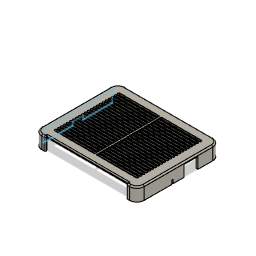
Grille (Autodesk Fusion 360 design; units mm, degrees)
Autodesk Fusion 360 part; units mm, degrees
sketch "Sketch1" plane through (0, 63.4, 0) normal (0, 1, 0) x (-1, 0, 0)
  line L0 (66.875, -54.475) -> (-66.875, -54.475)
  arc A0 (-68.875, -52.475) -> (-66.875, -54.475) centre (-66.875, -52.475) ccw
  line L1 (-68.875, -52.475) -> (-68.875, 52.475)
  arc A1 (-66.875, 54.475) -> (-68.875, 52.475) centre (-66.875, 52.475) ccw
  line L2 (-66.875, 54.475) -> (66.875, 54.475)
  arc A2 (68.875, 52.475) -> (66.875, 54.475) centre (66.875, 52.475) ccw
  line L3 (68.875, 52.475) -> (68.875, -52.475)
  arc A3 (66.875, -54.475) -> (68.875, -52.475) centre (66.875, -52.475) ccw
  line L4 (-66.4, -59.92) -> (66.4, -59.92)
  arc A4 (66.4, -59.92) -> (74.4, -51.92) centre (66.4, -51.92) ccw
  line L5 (74.4, -51.92) -> (74.4, 51.92)
  arc A5 (74.4, 51.92) -> (66.4, 59.92) centre (66.4, 51.92) ccw
  line L6 (66.4, 59.92) -> (-66.4, 59.92)
  arc A6 (-66.4, 59.92) -> (-74.4, 51.92) centre (-66.4, 51.92) ccw
  line L7 (-74.4, 51.92) -> (-74.4, -51.92)
  arc A7 (-74.4, -51.92) -> (-66.4, -59.92) centre (-66.4, -51.92) ccw
  line L8 (74.7, -51.92) -> (74.7, 51.92)
  arc A8 (74.7, 51.92) -> (66.4, 60.22) centre (66.4, 51.92) ccw
  line L9 (66.4, 60.22) -> (-66.4, 60.22)
  arc A9 (-66.4, 60.22) -> (-74.7, 51.92) centre (-66.4, 51.92) ccw
  line L10 (-74.7, 51.92) -> (-74.7, -51.92)
  arc A10 (-74.7, -51.92) -> (-66.4, -60.22) centre (-66.4, -51.92) ccw
  line L11 (-66.4, -60.22) -> (66.4, -60.22)
  arc A11 (66.4, -60.22) -> (74.7, -51.92) centre (66.4, -51.92) ccw
  line L12 (77.4, -51.92) -> (77.4, 51.92)
  arc A12 (77.4, 51.92) -> (66.4, 62.92) centre (66.4, 51.92) ccw
  line L13 (66.4, 62.92) -> (-66.4, 62.92)
  arc A13 (-66.4, 62.92) -> (-77.4, 51.92) centre (-66.4, 51.92) ccw
  line L14 (-77.4, 51.92) -> (-77.4, -51.92)
  arc A14 (-77.4, -51.92) -> (-66.4, -62.92) centre (-66.4, -51.92) ccw
  line L15 (-66.4, -62.92) -> (66.4, -62.92)
  arc A15 (66.4, -62.92) -> (77.4, -51.92) centre (66.4, -51.92) ccw
  dimension "d238" = 0.3
  dimension "d239" = 3
extrude "Extrude1" add sketch "Sketch1" against normal blind 17 contours L12 A12 L13 A13 L14 A14 L15 A15
extrude "Extrude2" add sketch "Sketch1" along normal blind 3 contours L0 A0 L1 A1 L2 A2 L3 A3 | L4 A4 L5 A5 L6 A6 L7 A7 | L8 A8 L9 A9 L10 A10 L11 A11 | L12 A12 L13 A13 L14 A14 L15 A15
sketch "Sketch2" plane through (0, 66.4, 0) normal (0, 1, 0) x (-1, 0, 0)
  line L0 (66.4, -59.92) -> (0, -59.92)
  line L1 (0, -59.92) -> (63, -59.92)
  line L2 (74.4, -51.92) -> (74.4, 0) construction
  line L3 (63, 0) -> (74.4, 0) construction
  line L4 (63, 0) -> (63, -48.5) construction
  line L5 (63, -48.5) -> (189, -48.5) construction
  line L6 (189, -48.5) -> (189, 48.5) construction
  line L7 (189, 48.5) -> (63, 48.5) construction
  line L8 (63, 48.5) -> (63, -48.5) construction
  line L9 (61.5, -47) -> (-61.5, -47)
  arc A0 (-61.5, -47) -> (-61.5, -50) centre (-61.5, -48.5) ccw
  line L10 (-61.5, -50) -> (61.5, -50)
  arc A1 (61.5, -50) -> (61.5, -47) centre (61.5, -48.5) ccw
  line L11 (63, -48.5) -> (-63, -48.5) construction
  line L12 (-61.5, -45.4762) -> (61.5, -45.4762)
  line L13 (61.5, -42.4762) -> (-61.5, -42.4762)
  arc A2 (61.5, -45.4762) -> (61.5, -42.4762) centre (61.5, -43.9762) ccw
  arc A3 (-61.5, -42.4762) -> (-61.5, -45.4762) centre (-61.5, -43.9762) ccw
  line L14 (-61.5, -40.9524) -> (61.5, -40.9524)
  line L15 (61.5, -37.9524) -> (-61.5, -37.9524)
  arc A4 (61.5, -40.9524) -> (61.5, -37.9524) centre (61.5, -39.4524) ccw
  arc A5 (-61.5, -37.9524) -> (-61.5, -40.9524) centre (-61.5, -39.4524) ccw
  line L16 (-61.5, -36.4286) -> (61.5, -36.4286)
  line L17 (61.5, -33.4286) -> (-61.5, -33.4286)
  arc A6 (61.5, -36.4286) -> (61.5, -33.4286) centre (61.5, -34.9286) ccw
  arc A7 (-61.5, -33.4286) -> (-61.5, -36.4286) centre (-61.5, -34.9286) ccw
  line L18 (-61.5, -31.9048) -> (61.5, -31.9048)
  line L19 (61.5, -28.9048) -> (-61.5, -28.9048)
  arc A8 (61.5, -31.9048) -> (61.5, -28.9048) centre (61.5, -30.4048) ccw
  arc A9 (-61.5, -28.9048) -> (-61.5, -31.9048) centre (-61.5, -30.4048) ccw
  line L20 (-61.5, -27.381) -> (61.5, -27.381)
  line L21 (61.5, -24.381) -> (-61.5, -24.381)
  arc A10 (61.5, -27.381) -> (61.5, -24.381) centre (61.5, -25.881) ccw
  arc A11 (-61.5, -24.381) -> (-61.5, -27.381) centre (-61.5, -25.881) ccw
  line L22 (-61.5, -22.8571) -> (61.5, -22.8571)
  line L23 (61.5, -19.8571) -> (-61.5, -19.8571)
  arc A12 (61.5, -22.8571) -> (61.5, -19.8571) centre (61.5, -21.3571) ccw
  arc A13 (-61.5, -19.8571) -> (-61.5, -22.8571) centre (-61.5, -21.3571) ccw
  line L24 (-61.5, -18.3333) -> (61.5, -18.3333)
  line L25 (61.5, -15.3333) -> (-61.5, -15.3333)
  arc A14 (61.5, -18.3333) -> (61.5, -15.3333) centre (61.5, -16.8333) ccw
  arc A15 (-61.5, -15.3333) -> (-61.5, -18.3333) centre (-61.5, -16.8333) ccw
  line L26 (-61.5, -13.8095) -> (61.5, -13.8095)
  line L27 (61.5, -10.8095) -> (-61.5, -10.8095)
  arc A16 (61.5, -13.8095) -> (61.5, -10.8095) centre (61.5, -12.3095) ccw
  arc A17 (-61.5, -10.8095) -> (-61.5, -13.8095) centre (-61.5, -12.3095) ccw
  line L28 (-61.5, -9.2857) -> (61.5, -9.2857)
  line L29 (61.5, -6.2857) -> (-61.5, -6.2857)
  arc A18 (61.5, -9.2857) -> (61.5, -6.2857) centre (61.5, -7.7857) ccw
  arc A19 (-61.5, -6.2857) -> (-61.5, -9.2857) centre (-61.5, -7.7857) ccw
  line L30 (-61.5, -4.7619) -> (61.5, -4.7619)
  line L31 (61.5, -1.7619) -> (-61.5, -1.7619)
  arc A20 (61.5, -4.7619) -> (61.5, -1.7619) centre (61.5, -3.2619) ccw
  arc A21 (-61.5, -1.7619) -> (-61.5, -4.7619) centre (-61.5, -3.2619) ccw
  line L32 (-61.5, -0.2381) -> (61.5, -0.2381)
  line L33 (61.5, 2.7619) -> (-61.5, 2.7619)
  arc A22 (61.5, -0.2381) -> (61.5, 2.7619) centre (61.5, 1.2619) ccw
  arc A23 (-61.5, 2.7619) -> (-61.5, -0.2381) centre (-61.5, 1.2619) ccw
  line L34 (-61.5, 4.2857) -> (61.5, 4.2857)
  line L35 (61.5, 7.2857) -> (-61.5, 7.2857)
  arc A24 (61.5, 4.2857) -> (61.5, 7.2857) centre (61.5, 5.7857) ccw
  arc A25 (-61.5, 7.2857) -> (-61.5, 4.2857) centre (-61.5, 5.7857) ccw
  line L36 (-61.5, 8.8095) -> (61.5, 8.8095)
  line L37 (61.5, 11.8095) -> (-61.5, 11.8095)
  arc A26 (61.5, 8.8095) -> (61.5, 11.8095) centre (61.5, 10.3095) ccw
  arc A27 (-61.5, 11.8095) -> (-61.5, 8.8095) centre (-61.5, 10.3095) ccw
  line L38 (-61.5, 13.3333) -> (61.5, 13.3333)
  line L39 (61.5, 16.3333) -> (-61.5, 16.3333)
  arc A28 (61.5, 13.3333) -> (61.5, 16.3333) centre (61.5, 14.8333) ccw
  arc A29 (-61.5, 16.3333) -> (-61.5, 13.3333) centre (-61.5, 14.8333) ccw
  line L40 (-61.5, 17.8571) -> (61.5, 17.8571)
  line L41 (61.5, 20.8571) -> (-61.5, 20.8571)
  arc A30 (61.5, 17.8571) -> (61.5, 20.8571) centre (61.5, 19.3571) ccw
  arc A31 (-61.5, 20.8571) -> (-61.5, 17.8571) centre (-61.5, 19.3571) ccw
  line L42 (-61.5, 22.381) -> (61.5, 22.381)
  line L43 (61.5, 25.381) -> (-61.5, 25.381)
  arc A32 (61.5, 22.381) -> (61.5, 25.381) centre (61.5, 23.881) ccw
  arc A33 (-61.5, 25.381) -> (-61.5, 22.381) centre (-61.5, 23.881) ccw
  line L44 (-61.5, 26.9048) -> (61.5, 26.9048)
  line L45 (61.5, 29.9048) -> (-61.5, 29.9048)
  arc A34 (61.5, 26.9048) -> (61.5, 29.9048) centre (61.5, 28.4048) ccw
  arc A35 (-61.5, 29.9048) -> (-61.5, 26.9048) centre (-61.5, 28.4048) ccw
  line L46 (-61.5, 31.4286) -> (61.5, 31.4286)
  line L47 (61.5, 34.4286) -> (-61.5, 34.4286)
  arc A36 (61.5, 31.4286) -> (61.5, 34.4286) centre (61.5, 32.9286) ccw
  arc A37 (-61.5, 34.4286) -> (-61.5, 31.4286) centre (-61.5, 32.9286) ccw
  line L48 (-61.5, 35.9524) -> (61.5, 35.9524)
  line L49 (61.5, 38.9524) -> (-61.5, 38.9524)
  arc A38 (61.5, 35.9524) -> (61.5, 38.9524) centre (61.5, 37.4524) ccw
  arc A39 (-61.5, 38.9524) -> (-61.5, 35.9524) centre (-61.5, 37.4524) ccw
  line L50 (-61.5, 40.4762) -> (61.5, 40.4762)
  line L51 (61.5, 43.4762) -> (-61.5, 43.4762)
  arc A40 (61.5, 40.4762) -> (61.5, 43.4762) centre (61.5, 41.9762) ccw
  arc A41 (-61.5, 43.4762) -> (-61.5, 40.4762) centre (-61.5, 41.9762) ccw
  line L52 (-61.5, 45) -> (61.5, 45)
  line L53 (61.5, 48) -> (-61.5, 48)
  arc A42 (61.5, 45) -> (61.5, 48) centre (61.5, 46.5) ccw
  arc A43 (-61.5, 48) -> (-61.5, 45) centre (-61.5, 46.5) ccw
  line L54 (0, -50) -> (1.5, -50)
  line L55 (1.5, -50) -> (-1.5, -50)
  line L56 (-1.5, -50) -> (-1.5, 48)
  line L57 (-1.5, 48) -> (1.5, 48)
  line L58 (1.5, 48) -> (1.5, -50)
  arc A44 (66.4, -62.92) -> (77.4, -51.92) centre (66.4, -51.92) ccw
  line L59 (77.4, -51.92) -> (77.4, 51.92)
  arc A45 (77.4, 51.92) -> (66.4, 62.92) centre (66.4, 51.92) ccw
  line L60 (66.4, 62.92) -> (-66.4, 62.92)
  arc A46 (-66.4, 62.92) -> (-77.4, 51.92) centre (-66.4, 51.92) ccw
  line L61 (-77.4, 51.92) -> (-77.4, -51.92)
  arc A47 (-77.4, -51.92) -> (-66.4, -62.92) centre (-66.4, -51.92) ccw
  line L62 (-66.4, -62.92) -> (66.4, -62.92)
  dimension "d244" = 63
  dimension "d246" = 48.5
  dimension "d247" = 126
  dimension "d248" = 97
  dimension "d249" = 126
  dimension "d250" = 3
  dimension "d253" = 0
  dimension "d254" = 95
  dimension "d257" = 1.5
  dimension "d258" = 3
  dimension "d259" = 98
  constraint coincident L0 L1.end
  constraint perpendicular L3 L4
  constraint horizontal L5
  constraint vertical L6
  constraint horizontal L7
  constraint vertical L8
  constraint tangent L9 A0
  constraint tangent A0 L10
  constraint parallel L9 L10
  constraint tangent L10 A1
  constraint tangent L9 A1
  constraint midpoint L4.end A1
  constraint midpoint A0 L11.end
  constraint perpendicular L4 L11
  constraint midpoint L10 L54.start
  constraint horizontal L54
  constraint horizontal L55
  constraint vertical L56
  constraint horizontal L57
  constraint vertical L58
  measures "d244" distance of L0.end L1.end
  measures "d246" distance of L3.start L4.end
  measures "d247" distance of L4.end L5.end
  measures "d248" distance of L4.end L7.end
  measures "d249" distance of L4.end L11.end
  measures "d250" diameter of A0
  measures "d257" distance of L54.start L54.end
  measures "d258" distance of L54.end L55.end
  measures "d259" distance of L54.end L57.end
extrude "Extrude3" cut sketch "Sketch2" against normal up to surface (3 mm away) contours L9 L10 A1 L58 | L9 A0 L10 L56 | L12 L13 A2 L58 | L12 L13 A3 L56 | L14 L15 A4 L58 | L14 L15 A5 L56 | L16 L17 A6 L58 | L16 L17 A7 L56 | L18 L19 A8 L58 | L18 L19 A9 L56 | L20 L21 A10 L58 | L20 L21 A11 L56 | L22 L23 A12 L58 | L22 L23 A13 L56 | L24 L25 A14 L58 | L24 L25 A15 L56 | L26 L27 A16 L58 | L26 L27 A17 L56 | L28 L29 A18 L58 | L28 L29 A19 L56 | L30 L31 A20 L58 | L30 L31 A21 L56 | L32 L33 A22 L58 | L32 L33 A23 L56 | L34 L35 A24 L58 | L34 L35 A25 L56 | L36 L37 A26 L58 | L36 L37 A27 L56 | L38 L39 A28 L58 | L38 L39 A29 L56 | L40 L41 A30 L58 | L40 L41 A31 L56 | L42 L43 A32 L58 | L42 L43 A33 L56 | L44 L45 A34 L58 | L44 L45 A35 L56 | L46 L47 A36 L58 | L46 L47 A37 L56 | L48 L49 A38 L58 | L48 L49 A39 L56 | L50 L51 A40 L58 | L50 L51 A41 L56 | L52 L53 A42 L58 | L52 L53 A43 L56
chamfer "Chamfer1" distance 0.7 angle 45 132 edges at (31.5, 63.4, 48) (63, 63.4, 46.5) (31.5, 63.4, 45) (31.5, 63.4, 43.4762) (63, 63.4, 41.9762) (31.5, 63.4, 40.4762) (31.5, 63.4, 38.9524) (63, 63.4, 37.4524) (31.5, 63.4, 35.9524) (31.5, 63.4, 34.4286) (63, 63.4, 32.9286) (31.5, 63.4, 31.4286) (31.5, 63.4, 29.9048) (63, 63.4, 28.4048) (31.5, 63.4, 26.9048) (31.5, 63.4, 25.381) (63, 63.4, 23.881) (31.5, 63.4, 22.381) (31.5, 63.4, 20.8571) (63, 63.4, 19.3571) (31.5, 63.4, 17.8571) (31.5, 63.4, 16.3333) (63, 63.4, 14.8333) (31.5, 63.4, 13.3333) (31.5, 63.4, 11.8095) (63, 63.4, 10.3095) (31.5, 63.4, 8.8095) (31.5, 63.4, 7.2857) (63, 63.4, 5.7857) (31.5, 63.4, 4.2857) (31.5, 63.4, 2.7619) (63, 63.4, 1.2619) (31.5, 63.4, -0.2381) (31.5, 63.4, -1.7619) (63, 63.4, -3.2619) (31.5, 63.4, -4.7619) (31.5, 63.4, -6.2857) (63, 63.4, -7.7857) (31.5, 63.4, -9.2857) (31.5, 63.4, -10.8095) (63, 63.4, -12.3095) (31.5, 63.4, -13.8095) (31.5, 63.4, -15.3333) (63, 63.4, -16.8333) (31.5, 63.4, -18.3333) (31.5, 63.4, -19.8571) (63, 63.4, -21.3571) (31.5, 63.4, -22.8571) (31.5, 63.4, -24.381) (63, 63.4, -25.881) (31.5, 63.4, -27.381) (31.5, 63.4, -28.9048) (63, 63.4, -30.4048) (31.5, 63.4, -31.9048) (31.5, 63.4, -33.4286) (63, 63.4, -34.9286) (31.5, 63.4, -36.4286) (31.5, 63.4, -37.9524) (63, 63.4, -39.4524) (31.5, 63.4, -40.9524) (31.5, 63.4, -42.4762) (63, 63.4, -43.9762) (31.5, 63.4, -45.4762) (31.5, 63.4, -47) (63, 63.4, -48.5) (31.5, 63.4, -50) (-31.5, 63.4, -50) (-63, 63.4, -48.5) (-31.5, 63.4, -47) (-31.5, 63.4, -45.4762) (-63, 63.4, -43.9762) (-31.5, 63.4, -42.4762) (-31.5, 63.4, -40.9524) (-63, 63.4, -39.4524) (-31.5, 63.4, -37.9524) (-31.5, 63.4, -36.4286) (-63, 63.4, -34.9286) (-31.5, 63.4, -33.4286) (-31.5, 63.4, -31.9048) (-63, 63.4, -30.4048) (-31.5, 63.4, -28.9048) (-31.5, 63.4, -27.381) (-63, 63.4, -25.881) (-31.5, 63.4, -24.381) (-31.5, 63.4, -22.8571) (-63, 63.4, -21.3571) (-31.5, 63.4, -19.8571) (-31.5, 63.4, -18.3333) (-63, 63.4, -16.8333) (-31.5, 63.4, -15.3333) (-31.5, 63.4, -13.8095) (-63, 63.4, -12.3095) (-31.5, 63.4, -10.8095) (-31.5, 63.4, -9.2857) (-63, 63.4, -7.7857) (-31.5, 63.4, -6.2857) (-31.5, 63.4, -4.7619) (-63, 63.4, -3.2619) (-31.5, 63.4, -1.7619) (-31.5, 63.4, -0.2381) (-63, 63.4, 1.2619) (-31.5, 63.4, 2.7619) (-31.5, 63.4, 4.2857) (-63, 63.4, 5.7857) (-31.5, 63.4, 7.2857) (-31.5, 63.4, 8.8095) (-63, 63.4, 10.3095) (-31.5, 63.4, 11.8095) (-31.5, 63.4, 13.3333) (-63, 63.4, 14.8333) (-31.5, 63.4, 16.3333) (-31.5, 63.4, 17.8571) (-63, 63.4, 19.3571) (-31.5, 63.4, 20.8571) (-31.5, 63.4, 22.381) (-63, 63.4, 23.881) (-31.5, 63.4, 25.381) (-31.5, 63.4, 26.9048) (-63, 63.4, 28.4048) (-31.5, 63.4, 29.9048) (-31.5, 63.4, 31.4286) (-63, 63.4, 32.9286) (-31.5, 63.4, 34.4286) (-31.5, 63.4, 35.9524) (-63, 63.4, 37.4524) (-31.5, 63.4, 38.9524) (-31.5, 63.4, 40.4762) (-63, 63.4, 41.9762) (-31.5, 63.4, 43.4762) (-31.5, 63.4, 45) (-63, 63.4, 46.5) (-31.5, 63.4, 48)
fillet "Fillet1" radius 0.3 176 edges at (31.5, 66.4, -45.4762) (63, 66.4, -43.9762) (31.5, 66.4, -42.4762) (1.5, 66.4, 19.3571) (31.5, 66.4, -27.381) (63, 66.4, -25.881) (31.5, 66.4, -24.381) (31.5, 66.4, -0.2381) (63, 66.4, 1.2619) (31.5, 66.4, 2.7619) (31.5, 66.4, -18.3333) (63, 66.4, -16.8333) (31.5, 66.4, -15.3333) (-31.5, 66.4, -19.8571) (-63, 66.4, -21.3571) (-31.5, 66.4, -22.8571) (31.5, 66.4, -36.4286) (63, 66.4, -34.9286) (31.5, 66.4, -33.4286) (1.5, 66.4, -39.4524) (31.5, 66.4, -22.8571) (63, 66.4, -21.3571) (31.5, 66.4, -19.8571) (1.5, 66.4, -34.9286) (1.5, 66.4, 14.8333) (-1.5, 66.4, -34.9286) (31.5, 66.4, -9.2857) (63, 66.4, -7.7857) (31.5, 66.4, -6.2857) (31.5, 66.4, 22.381) (63, 66.4, 23.881) (31.5, 66.4, 25.381) (-31.5, 66.4, -24.381) (-63, 66.4, -25.881) (-31.5, 66.4, -27.381) (31.5, 66.4, -13.8095) (63, 66.4, -12.3095) (31.5, 66.4, -10.8095) (31.5, 66.4, -50) (63, 66.4, -48.5) (31.5, 66.4, -47) (-31.5, 66.4, 2.7619) (-63, 66.4, 1.2619) (-31.5, 66.4, -0.2381) (31.5, 66.4, 35.9524) (63, 66.4, 37.4524) (31.5, 66.4, 38.9524) (-1.5, 66.4, 32.9286) (1.5, 66.4, -7.7857) (1.5, 66.4, 37.4524) (31.5, 66.4, 40.4762) (63, 66.4, 41.9762) (31.5, 66.4, 43.4762) (31.5, 66.4, 31.4286) (63, 66.4, 32.9286) (31.5, 66.4, 34.4286) (-31.5, 66.4, 43.4762) (-63, 66.4, 41.9762) (-31.5, 66.4, 40.4762) (-31.5, 66.4, -15.3333) (-63, 66.4, -16.8333) (-31.5, 66.4, -18.3333) (-31.5, 66.4, 48) (-63, 66.4, 46.5) (-31.5, 66.4, 45) (31.5, 66.4, 45) (63, 66.4, 46.5) (31.5, 66.4, 48) (-31.5, 66.4, 38.9524) (-63, 66.4, 37.4524) (-31.5, 66.4, 35.9524) (1.5, 66.4, -12.3095) (-1.5, 66.4, -12.3095) (-1.5, 66.4, -3.2619) (-31.5, 66.4, 11.8095) (-63, 66.4, 10.3095) (-31.5, 66.4, 8.8095) (1.5, 66.4, 32.9286) (1.5, 66.4, 46.5) (-31.5, 66.4, -37.9524) (-63, 66.4, -39.4524) (-31.5, 66.4, -40.9524) (-31.5, 66.4, 34.4286) (-63, 66.4, 32.9286) (-31.5, 66.4, 31.4286) (-31.5, 66.4, 16.3333) (-63, 66.4, 14.8333) (-31.5, 66.4, 13.3333) (-1.5, 66.4, 37.4524) (1.5, 66.4, 1.2619) (-1.5, 66.4, 5.7857) (-31.5, 66.4, -6.2857) (-63, 66.4, -7.7857) (-31.5, 66.4, -9.2857) (31.5, 66.4, -4.7619) (63, 66.4, -3.2619) (31.5, 66.4, -1.7619) (-31.5, 66.4, -10.8095) (-63, 66.4, -12.3095) (-31.5, 66.4, -13.8095) (-1.5, 66.4, 1.2619) (-1.5, 66.4, 19.3571) (31.5, 66.4, -31.9048) (63, 66.4, -30.4048) (31.5, 66.4, -28.9048) (-31.5, 66.4, -42.4762) (-63, 66.4, -43.9762) (-31.5, 66.4, -45.4762) (-31.5, 66.4, -47) (-63, 66.4, -48.5) (-31.5, 66.4, -50) (-31.5, 66.4, -28.9048) (-63, 66.4, -30.4048) (-31.5, 66.4, -31.9048) (-1.5, 66.4, 14.8333) (-1.5, 66.4, -39.4524) (-31.5, 66.4, 29.9048) (-63, 66.4, 28.4048) (-31.5, 66.4, 26.9048) (-31.5, 66.4, 20.8571) (-63, 66.4, 19.3571) (-31.5, 66.4, 17.8571) (31.5, 66.4, 4.2857) (63, 66.4, 5.7857) (31.5, 66.4, 7.2857) (31.5, 66.4, 8.8095) (63, 66.4, 10.3095) (31.5, 66.4, 11.8095) (31.5, 66.4, 17.8571) (63, 66.4, 19.3571) (31.5, 66.4, 20.8571) (1.5, 66.4, 23.881) (-1.5, 66.4, 23.881) (-1.5, 66.4, -48.5) (31.5, 66.4, 26.9048) (63, 66.4, 28.4048) (31.5, 66.4, 29.9048) (1.5, 66.4, -48.5) (31.5, 66.4, -40.9524) (63, 66.4, -39.4524) (31.5, 66.4, -37.9524) (1.5, 66.4, -43.9762) (-31.5, 66.4, 25.381) (-63, 66.4, 23.881) (-31.5, 66.4, 22.381) (-31.5, 66.4, 7.2857) (-63, 66.4, 5.7857) (-31.5, 66.4, 4.2857) (-1.5, 66.4, -25.881) (-1.5, 66.4, -7.7857) (1.5, 66.4, -3.2619) (31.5, 66.4, 13.3333) (63, 66.4, 14.8333) (31.5, 66.4, 16.3333) (1.5, 66.4, 5.7857) (-31.5, 66.4, -33.4286) (-63, 66.4, -34.9286) (-31.5, 66.4, -36.4286) (-31.5, 66.4, -1.7619) (-63, 66.4, -3.2619) (-31.5, 66.4, -4.7619) (1.5, 66.4, 10.3095) (-1.5, 66.4, -30.4048) (1.5, 66.4, 41.9762) (1.5, 66.4, -30.4048) (-1.5, 66.4, 41.9762) (-1.5, 66.4, 46.5) (-1.5, 66.4, 10.3095) (1.5, 66.4, 28.4048) (1.5, 66.4, -16.8333) (-1.5, 66.4, -21.3571) (-1.5, 66.4, -43.9762) (1.5, 66.4, -21.3571) (-1.5, 66.4, 28.4048) (-1.5, 66.4, -16.8333) (1.5, 66.4, -25.881)
sketch "Sketch3" plane through (77.4, 0, 0) normal (1, 0, 0) x (0, 0, -1)
  line L0 (-51.92, 66.4) -> (-51.92, 46.4)
  line L1 (-51.92, 46.4) -> (51.92, 46.4)
  line L2 (51.92, 46.4) -> (51.92, 66.4)
  line L3 (51.92, 66.4) -> (-51.92, 66.4)
  line L4 (51.92, 66.4) -> (51.92, 46.4)
  line L5 (51.92, 46.4) -> (62.92, 46.4)
  line L6 (62.92, 46.4) -> (62.92, 66.4)
  line L7 (62.92, 66.4) -> (51.92, 66.4)
  line L8 (62.92, 63.4) -> (51.92, 63.4)
  line L9 (-51.92, 63.4) -> (51.92, 63.4)
  line L10 (-62.92, 66.4) -> (-62.92, 46.4)
  line L11 (-62.92, 46.4) -> (-51.92, 46.4)
  line L12 (-51.92, 46.4) -> (-51.92, 66.4)
  line L13 (-51.92, 66.4) -> (-62.92, 66.4)
  line L14 (62.92, 63.4) -> (8.42, 63.4)
  line L15 (8.42, 63.4) -> (29.42, 63.4)
  line L16 (29.42, 63.4) -> (29.42, 46.4)
  line L17 (29.42, 46.4) -> (8.42, 46.4)
  line L18 (8.42, 46.4) -> (8.42, 63.4)
  dimension "d262" = 54.5
  dimension "d263" = 21
  dimension "d264" = 17
  constraint coincident L8.start L14.start
  constraint perpendicular L2 L14
  constraint horizontal L15
  constraint vertical L16
  constraint horizontal L17
  constraint vertical L18
  measures "d262" distance of L8.start L14.end
  measures "d263" distance of L14.end L15.end
  measures "d264" distance of L14.end L17.end
extrude "Extrude4" cut sketch "Sketch3" against normal up to surface (2.7 mm away) contours L1 L9 L14 L15 L16 L17 L18
fillet "Fillet2" radius 2 8 edges at (-74.1782, 66.4, 59.6982) (0, 66.4, 62.92) (74.1782, 66.4, 59.6982) (77.4, 66.4, 0) (74.1782, 66.4, -59.6982) (0, 66.4, -62.92) (-74.1782, 66.4, -59.6982) (-77.4, 66.4, 0)
sketch "Sketch4" plane through (0, 46.4, 0) normal (0, -1, 0) x (1, 0, 0)
  line L0 (77.4, -29.42) -> (74.7, -29.42)
  line L1 (74.7, -29.42) -> (74.7, -51.92)
  arc A0 (66.4, -60.22) -> (74.7, -51.92) centre (66.4, -51.92) ccw
  line L2 (66.4, -60.22) -> (-66.4, -60.22)
  arc A1 (-74.7, -51.92) -> (-66.4, -60.22) centre (-66.4, -51.92) ccw
  line L3 (-74.7, -51.92) -> (-74.7, 51.92)
  arc A2 (-66.4, 60.22) -> (-74.7, 51.92) centre (-66.4, 51.92) ccw
  line L4 (-66.4, 60.22) -> (66.4, 60.22)
  arc A3 (74.7, 51.92) -> (66.4, 60.22) centre (66.4, 51.92) ccw
  line L5 (74.7, 51.92) -> (74.7, -8.42)
  line L6 (74.7, -8.42) -> (77.4, -8.42)
  line L7 (77.4, -8.42) -> (77.4, 51.92)
  arc A4 (77.4, 51.92) -> (66.4, 62.92) centre (66.4, 51.92) ccw
  line L8 (66.4, 62.92) -> (-66.4, 62.92)
  arc A5 (-66.4, 62.92) -> (-77.4, 51.92) centre (-66.4, 51.92) ccw
  line L9 (-77.4, 51.92) -> (-77.4, -51.92)
  arc A6 (-77.4, -51.92) -> (-66.4, -62.92) centre (-66.4, -51.92) ccw
  line L10 (-66.4, -62.92) -> (66.4, -62.92)
  arc A7 (66.4, -62.92) -> (77.4, -51.92) centre (66.4, -51.92) ccw
  line L11 (77.4, -51.92) -> (77.4, -29.42)
  line L12 (0, 62.92) -> (-77.4, 62.92)
  line L13 (-77.4, 62.92) -> (-61.4, 62.92)
  line L14 (0, 62.92) -> (77.4, 62.92)
  line L15 (77.4, 62.92) -> (61.4, 62.92)
  line L16 (-61.4, 62.92) -> (61.4, 62.92)
  line L17 (61.4, 62.92) -> (61.4, 60.22)
  line L18 (61.4, 60.22) -> (-61.4, 60.22)
  line L19 (-61.4, 60.22) -> (-61.4, 62.92)
  dimension "d469" = 16
  dimension "d470" = 16
  constraint midpoint L8 L12.start
  constraint perpendicular L9 L12
  constraint perpendicular L9 L13
  constraint perpendicular L7 L14
  constraint parallel L14 L15
  constraint horizontal L16
  constraint vertical L17
  constraint horizontal L18
  constraint vertical L19
  constraint coincident L4 L17.end
  measures "d469" distance of L12.end L13.end
  measures "d470" distance of L14.end L15.end
extrude "Extrude5" cut sketch "Sketch4" against normal blind 20 contours L4 L8 L12 L14 L16 L17 L18 L19
fillet "Fillet3" radius 1.5 7 edges at (-61.4, 55.4, 62.92) (-61.4, 65.8142, 62.3342) (-61.4, 66.4, 60.57) (0, 66.4, 60.22) (61.4, 66.4, 60.57) (61.4, 65.8142, 62.3342) (61.4, 55.4, 62.92)
sketch "Sketch5" plane through (-74.7, 0, 0) normal (1, 0, 0) x (0, 0, -1)
  line L0 (8, 51.4) -> (-8, 51.4)
  line L1 (-8, 51.4) -> (-8, 41.4)
  line L2 (8, 41.4) -> (8, 51.4)
  line L3 (-51.92, 46.4) -> (51.92, 46.4)
extrude "Extrude6" add sketch "Sketch5" along normal blind 0.26
chamfer "Chamfer2" distance 2 distance2 0.2 1 edges at (-74.44, 51.4, 0) measured on face at (-74.44, 49.7333, 2.6667)
chamfer "Chamfer3" distance 2 distance2 0.2 1 edges at (-74.44, 46.4, 0) measured on face at (-74.44, 48.4, 2.6667)
sketch "Sketch6" plane through (74.7, 0, 0) normal (-1, 0, 0) x (0, 0, 1)
  line L0 (-8.42, 63.4) -> (-8.42, 46.4)
  line L1 (-8.42, 46.4) -> (51.92, 46.4)
  line L2 (51.92, 46.4) -> (51.92, 63.4)
  line L3 (51.92, 63.4) -> (-8.42, 63.4)
  line L4 (-8, 51.4) -> (8, 51.4)
  line L5 (-8, 41.4) -> (-8, 51.4)
  line L6 (8, 51.4) -> (8, 41.4)
  line L7 (51.92, 46.4) -> (-8.42, 46.4)
extrude "Extrude7" add sketch "Sketch6" along normal blind 0.26 contours L1 L4 L5 L6 L7
chamfer "Chamfer4" distance 2 distance2 0.2 1 edges at (74.44, 51.4, 0) measured on face at (74.44, 48.0667, 2.6667)
chamfer "Chamfer5" distance 2 distance2 0.2 1 edges at (74.44, 46.4, 0) measured on face at (74.44, 48.4, -2.6667)
sketch "Sketch7" plane through (0, 46.4, 0) normal (0, -1, 0) x (1, 0, 0)
  line L0 (-74.64, -8) -> (-74.64, 8)
  line L1 (-74.64, 8) -> (-74.7, 8)
  line L2 (-74.7, 8) -> (-74.7, 51.92)
  arc A0 (-66.4, 60.22) -> (-74.7, 51.92) centre (-66.4, 51.92) ccw
  line L3 (-66.4, 60.22) -> (-61.4, 60.22)
  line L4 (-61.4, 60.22) -> (-61.4, 61.42)
  arc A1 (-61.4, 61.42) -> (-62.9, 62.92) centre (-62.9, 61.42) ccw
  line L5 (-62.9, 62.92) -> (-66.4, 62.92)
  arc A2 (-66.4, 62.92) -> (-77.4, 51.92) centre (-66.4, 51.92) ccw
  line L6 (-77.4, 51.92) -> (-77.4, -51.92)
  arc A3 (-77.4, -51.92) -> (-66.4, -62.92) centre (-66.4, -51.92) ccw
  line L7 (-66.4, -62.92) -> (66.4, -62.92)
  arc A4 (66.4, -62.92) -> (77.4, -51.92) centre (66.4, -51.92) ccw
  line L8 (77.4, -51.92) -> (77.4, -29.42)
  line L9 (77.4, -29.42) -> (74.7, -29.42)
  line L10 (74.7, -29.42) -> (74.7, -51.92)
  arc A5 (66.4, -60.22) -> (74.7, -51.92) centre (66.4, -51.92) ccw
  line L11 (66.4, -60.22) -> (-66.4, -60.22)
  arc A6 (-74.7, -51.92) -> (-66.4, -60.22) centre (-66.4, -51.92) ccw
  line L12 (-74.7, -51.92) -> (-74.7, -8)
  line L13 (-74.7, -8) -> (-74.64, -8)
  line L14 (-77.4, 51.92) -> (-77.4, -51.92)
  line L15 (77.4, -8.42) -> (77.4, 51.92)
  line L16 (-74.7, 8) -> (-77.4, 8)
  line L17 (-77.4, 8) -> (-77.4, 10)
  line L18 (-77.4, 10) -> (-74.7, 10)
  line L19 (-74.7, 10) -> (-74.7, 8)
  line L20 (-74.7, -8) -> (-77.4, -8)
  line L21 (-77.4, -8) -> (-77.4, -10)
  line L22 (-77.4, -10) -> (-74.7, -10)
  line L23 (-74.7, -10) -> (-74.7, -8)
  line L24 (74.7, 8) -> (77.4, 8)
  line L25 (77.4, 8) -> (77.4, 10)
  line L26 (77.4, 10) -> (74.7, 10)
  line L27 (74.7, 10) -> (74.7, 8)
  point P0 (-74.7, 8)
  point P1 (-74.7, -8)
  point P2 (74.7, 8)
  point P3 (74.7, -8)
  dimension "d488" = 2
  dimension "d489" = 2
  dimension "d490" = 2
  constraint horizontal L16
  constraint vertical L17
  constraint horizontal L18
  constraint vertical L19
  constraint coincident P0 L1.end
  constraint horizontal L20
  constraint vertical L21
  constraint horizontal L22
  constraint vertical L23
  constraint coincident P1 L12.end
  constraint horizontal L24
  constraint vertical L25
  constraint horizontal L26
  constraint vertical L27
  constraint coincident P2 L24.start
  measures "d488" distance of P0 L18.end
  measures "d489" distance of P1 L22.end
  measures "d490" distance of P2 L26.end
extrude "Extrude8" cut sketch "Sketch7" against normal blind 6 contours L6 L12 L14 L20 L21 L22 L23 | L2 L6 L14 L16 L17 L18 L19 | L15 L24 L25 L26 L27
fillet "Fillet4" radius 1 6 edges at (-76.05, 52.4, 10) (-76.05, 52.4, 8) (-76.05, 52.4, -10) (76.05, 52.4, 8) (76.05, 52.4, 10) (-76.05, 52.4, -8)
